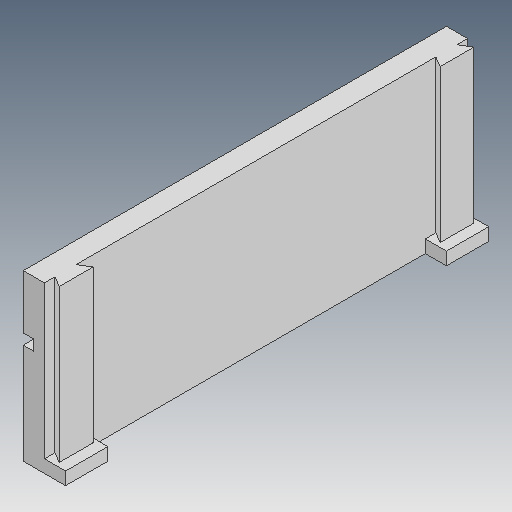
# Autodesk Inventor part: drawersidehalf
Saved by Autodesk Inventor 2025.2 (Build 292293000, 293)
## iProperties
Created: 2025-02-24
Part Number: drawersidehalf
Material: Generic
Document SubType Name: Modeling
Designer: email
Density: 1 g/cm^3
Appearance: Default
Author: email
Autodesk Inventor part; units mm, degrees
ref_plane "YZ Plane" through (0, 0, 0) normal (1, 0, 0) x (0, 1, 0)
ref_plane "XZ Plane" through (0, 0, 0) normal (0, 1, 0) x (-1, 0, 0)
ref_plane "XY Plane" through (0, 0, 0) normal (0, 0, 1) x (1, 0, 0)
sketch "Sketch1" plane through (0, 0, 0) normal (0, 1, 0) x (-1, 0, 0)
  line L0 (0, 0) -> (0, -100)
  line L1 (0, -100) -> (-5, -100)
  line L2 (-5, -100) -> (-5, -97.5)
  line L3 (-5, -92.5) -> (-5, -7.5)
  line L4 (-5, -7.5) -> (-7.5, -9)
  line L5 (-7.5, -9) -> (-7.5, -1)
  line L6 (-7.5, -1) -> (-5, -2.5)
  line L7 (-5, -2.5) -> (-5, 0)
  line L8 (-5, 0) -> (0, 0)
  line L9 (-5, -7.5) -> (-5, -2.5) construction
  line L10 (-5, -92.5) -> (-5, -97.5) construction
  line L11 (0, -50) -> (-5, -50) construction
  line L12 (-5, -92.5) -> (-7.5, -91)
  line L13 (-7.5, -91) -> (-7.5, -99)
  line L14 (-7.5, -99) -> (-5, -97.5)
  line L15 (0, 0) -> (-10, 0)
  line L16 (-10, 0) -> (-10, -10)
  line L17 (-10, -10) -> (0, -10)
  line L18 (0, -10) -> (0, 0)
  line L19 (0, -100) -> (-10, -100)
  line L20 (-10, -100) -> (-10, -90)
  line L21 (-10, -90) -> (0, -90)
  line L22 (0, -90) -> (0, -100)
  point P0 (-7.5, -5)
  point P1 (-5, -5)
  point P2 (-5, -95)
  point P3 (0, -90)
  point P4 (-5, 0)
  point P5 (0, -10)
  point P6 (-5, -90)
  dimension "d0" = 100
  dimension "d1" = 5
  dimension "d2" = 8
  dimension "d3" = 5
  dimension "d4" = 5
  dimension "d5" = 2.5
  dimension "d6" = 5
  dimension "d9" = 5
  dimension "d10" = 10
  dimension "d11" = 10
  dimension "d12" = 10
  dimension "d13" = 10
  constraints: 46 end point, 5 midpoint, 5 parallel, 5 perpendicular, 4 vertical, 2 horizontal, 2 point on line, 2 symmetric about line, 1 collinear, 1 horizontal alignment
  measures "d0" distance between parallel lines of L1 L8
  measures "d1" distance between parallel lines of L0 L3
  measures "d2" distance of L4.end L5.end
  measures "d3" distance of L6.end L3.end
  measures "d4" distance from line of L8 point (-7.5, -5)
  measures "d5" distance between parallel lines of L7 L5
  measures "d6" distance of L3.start L2.end
  measures "d9" distance from line of L1 point (-5, -95)
  measures "d10" distance of L0.start L15.end
  measures "d11" distance of L15.end L16.end
  measures "d12" distance of L20.end L21.end
  measures "d13" distance of L19.end L20.end
extrude "Extrusion1" add sketch "Sketch1" along normal blind 3 contours L0 L17 L3 L4 L5 L6 L7 L8 | L7 L6 L5 L4 L3 L17 L16 L15 | L0 L1 L2 L14 L13 L12 L3 L21 | L3 L12 L13 L14 L2 L19 L20 L21
extrude "Extrusion2" add sketch "Sketch1" along normal blind 39 contours L0 L17 L3 L4 L5 L6 L7 L8 | L0 L21 L3 L17 | L0 L1 L2 L14 L13 L12 L3 L21
sketch "Sketch2" plane through (0, 0, 0) normal (0, 0, 1) x (1, 0, 0)
  line L0 (0, 0) -> (0, 39) projected
  line L1 (0, 23.75) -> (2.5, 23.75)
  line L2 (2.5, 23.75) -> (2.5, 26.25)
  line L3 (2.5, 26.25) -> (0, 26.25)
  line L4 (0, 26.25) -> (0, 23.75)
  line L5 (0, 0) -> (10, 0) projected
  point P0 (0, 25.25)
  point P1 (2.5, 32.75)
  point P2 (2.5, 25)
  point P3 (0, 26.25)
  dimension "d21" = 25
  dimension "d22" = 2.5
  constraints: 8 end point, 3 point on line, 2 parallel, 1 horizontal, 1 midpoint, 1 perpendicular
  measures "d21" distance from line of L5 point (2.5, 25)
  measures "d22" distance between parallel lines of L1 L3
extrude "Extrusion3" cut sketch "Sketch2" against normal up to surface (100 mm away)
body "Solid1"
